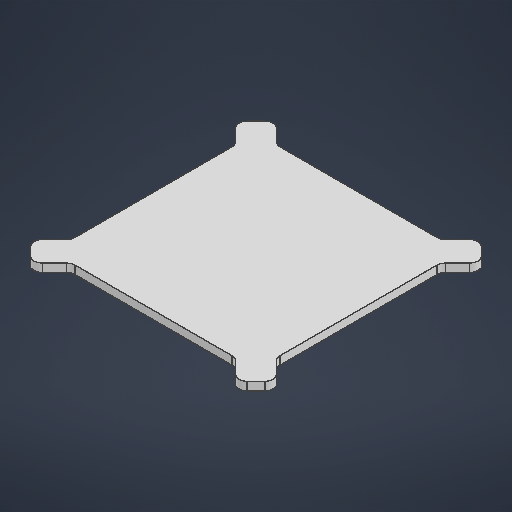
# Autodesk Inventor part: drone
Saved by Autodesk Inventor 2026 (Build 300175050, 175E)
## iProperties
Created: 2026-01-18
Part Number: drone
Material: Generic
Document SubType Name: Modeling
Designer: anawa
Density: 1 g/cm^3
Appearance: Default
Author: anawa
Autodesk Inventor part; units mm, degrees
ref_plane "YZ Plane" through (0, 0, 0) normal (1, 0, 0) x (0, 1, 0)
ref_plane "XZ Plane" through (0, 0, 0) normal (0, 1, 0) x (-1, 0, 0)
ref_plane "XY Plane" through (0, 0, 0) normal (0, 0, 1) x (1, 0, 0)
sketch "Sketch1" plane through (0, 0, 0) normal (0, 1, 0) x (-1, 0, 0)
  line L0 (-25, 25) -> (25, 25)
  line L1 (25, 25) -> (25, -25)
  line L2 (25, -25) -> (-25, -25)
  line L3 (-25, -25) -> (-25, 25)
  line L4 (-25, 25) -> (25, -25) construction
  line L5 (25, 25) -> (-25, -25) construction
  line L6 (-30, 30) -> (30, 30) construction
  line L7 (30, 30) -> (30, -30) construction
  line L8 (30, -30) -> (-30, -30) construction
  line L9 (-30, -30) -> (-30, 30) construction
  line L10 (-30, 30) -> (30, -30) construction
  line L11 (30, 30) -> (-30, -30) construction
  line L12 (-25, 30) -> (-30, 25)
  line L13 (-30, 25) -> (-25, 30)
  line L14 (-25, 30) -> (-20, 25)
  line L15 (-20, 25) -> (-25, 20)
  line L16 (-25, 20) -> (-30, 25)
  line L17 (0, 0) -> (0, 2.49) construction
  line L18 (0, 0) -> (2.0714, 0) construction
  line L19 (25, 30) -> (30, 25)
  line L20 (25, 30) -> (20, 25)
  line L21 (20, 25) -> (25, 20)
  line L22 (25, 20) -> (30, 25)
  line L23 (-25, -30) -> (-30, -25)
  line L24 (-25, -30) -> (-20, -25)
  line L25 (-20, -25) -> (-25, -20)
  line L26 (-25, -20) -> (-30, -25)
  line L27 (25, -30) -> (20, -25)
  line L28 (25, -20) -> (30, -25)
  line L29 (25, -30) -> (30, -25)
  line L30 (20, -25) -> (25, -20)
  dimension "d0" = 50
  dimension "d1" = 50
  dimension "d2" = 60
  dimension "d3" = 60
  dimension "d4" = 5
  dimension "d5" = 5
  constraints: 62 end point, 12 symmetric about line, 7 equal length, 4 midpoint, 3 horizontal, 3 perpendicular, 2 point on line, 1 vertical
  measures "d0" distance of L0.end L1.end
  measures "d1" distance of L1.end L2.end
  measures "d2" distance of L6.end L7.end
  measures "d3" distance of L7.end L8.end
  measures "d4" distance of L6.start L12.start
  measures "d5" distance of L6.start L12.end
extrude "Extrusion1" add sketch "Sketch1" along normal blind 2
fillet "Fillet1" radius 2 16 edges at (30, 1, 25) (25, 1, 30) (25, 1, 20) (25, 1, -20) (30, 1, -25) (25, 1, -30) (20, 1, -25) (-20, 1, -25) (-25, 1, -30) (-30, 1, -25) (-25, 1, -20) (-25, 1, 20) (-20, 1, 25) (-30, 1, 25) (-25, 1, 30) (20, 1, 25)
body "Solid1"
